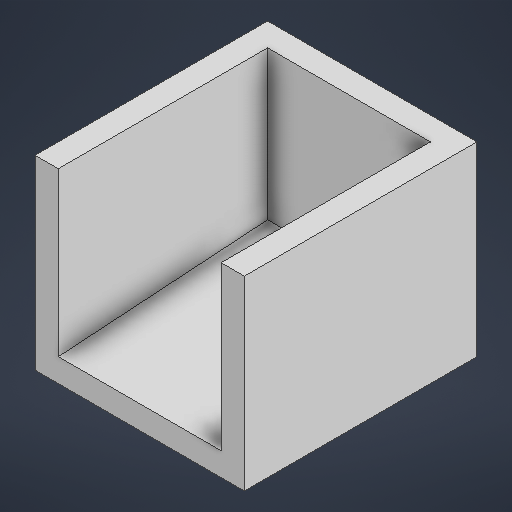
# Autodesk Inventor part: outstorage
Saved by Autodesk Inventor 2026.2 (Build 302298000, 298)
## iProperties
Created: 2026-04-16
Part Number: outstorage
Material: Generic
Document SubType Name: Modeling
Designer: danda
Density: 1 g/cm^3
Appearance: Default
Author: danda
Autodesk Inventor part; units mm, degrees
ref_plane "YZ Plane" through (0, 0, 0) normal (1, 0, 0) x (0, 1, 0)
ref_plane "XZ Plane" through (0, 0, 0) normal (0, 1, 0) x (-1, 0, 0)
ref_plane "XY Plane" through (0, 0, 0) normal (0, 0, 1) x (1, 0, 0)
sketch "Sketch1" plane through (0, 0, 0) normal (0, 0, 1) x (1, 0, 0)
  line L0 (22.7313, 23.816) -> (22.7313, -11.184)
  line L1 (22.7313, -11.184) -> (57.7313, -11.184)
  line L2 (57.7313, -11.184) -> (57.7313, 23.816)
  line L3 (17.7313, 23.816) -> (17.7313, -16.184)
  line L4 (17.7313, -16.184) -> (62.7313, -16.184)
  line L5 (62.7313, -16.184) -> (62.7313, 23.816)
  line L6 (17.7313, 23.816) -> (22.7313, 23.816)
  line L7 (57.7313, 23.816) -> (62.7313, 23.816)
  line L8 (17.7313, 23.816) -> (62.7313, 23.816)
  point P0 (0, 0)
  point P1 (57.7313, 23.816)
  dimension "d0" = 35
  dimension "d1" = 35
  dimension "d2" = 35
  dimension "d3" = 5
  constraints: 18 end point, 2 parallel, 2 perpendicular, 1 horizontal, 1 vertical, 2 other
  measures "d0" distance of L0.start L0.end
  measures "d1" distance of L0.end L1.end
  measures "d2" distance of L1.end L2.end
  measures "d3" distance between parallel lines of L0 L3
extrude "Extrusion1" add sketch "Sketch1" along normal blind 5
extrude "Extrusion2" add sketch "Sketch1" along normal blind 50 contours L0 L1 L2 L7 L5 L4 L3 L6
sketch "Sketch2" plane through (57.7313, -11.184, 5) normal (-1, 0, 0) x (0, 0, 1)
  line L0 (0, 35) -> (0, 0) projected
  line L1 (0, 0) -> (0, 3)
  line L2 (0, 0) -> (45, 0) projected
  line L3 (0, 3) -> (45, 0)
  line L4 (45, 0) -> (0, 3)
  point P0 (-5, 11.184)
  dimension "d8" = 3
  constraints: 6 end point, 1 collinear, 1 point on line
  measures "d8" distance of L0.end L1.end
extrude "Extrusion3" add sketch "Sketch2" along normal blind 35
body "Solid1"
